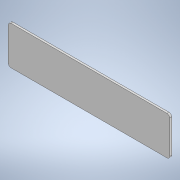
# Autodesk Inventor part: back_panel
Saved by Autodesk Inventor 2021 (Build 250183000, 183)
## iProperties
Created: 2026-03-01
Part Number: back_panel
Material: Generic
Document SubType Name: Modeling
Designer: Toby
Density: 1 g/cm^3
Appearance: Default
Author: Toby
Autodesk Inventor part; units mm, degrees
ref_plane "YZ Plane" through (0, 0, 0) normal (1, 0, 0) x (0, 1, 0)
ref_plane "XZ Plane" through (0, 0, 0) normal (0, 1, 0) x (-1, 0, 0)
ref_plane "XY Plane" through (0, 0, 0) normal (0, 0, 1) x (1, 0, 0)
sketch "Sketch1" plane through (0, 0, 0) normal (0, 0, 1) x (1, 0, 0)
  line L0 (-59.9, 14.1) -> (60.3, 14.1)
  line L1 (60.3, 14.1) -> (60.3, -14.6)
  line L2 (60.3, -14.6) -> (-59.9, -14.6)
  line L3 (-59.9, -14.6) -> (-59.9, 14.1)
  point P0 (0, 0)
  dimension "d0" = 120.2
  dimension "d1" = 28.7
  dimension "d2" = 59.9
  dimension "d3" = 14.1
  constraints: 8 end point, 2 parallel, 1 horizontal, 1 perpendicular
  measures "d0" distance of L0.start L0.end
  measures "d1" distance of L2.end L0.start
  measures "d2" distance from line of point (0, 0) L3
  measures "d3" distance from line of point (0, 0) L0
extrude "Extrusion1" add sketch "Sketch1" along normal blind 1.5
fillet "Fillet1" radius 2 4 edges at (-59.9, 14.1, 0.75) (60.3, 14.1, 0.75) (60.3, -14.6, 0.75) (-59.9, -14.6, 0.75)
body "Solid1"
